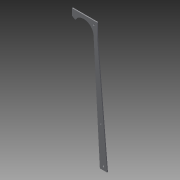
# Autodesk Inventor part: PassiveHooks2
Saved by Autodesk Inventor 2013 (Build 170138000, 138)
## iProperties
Created: 2013-02-07
Part Number: PassiveHooks2
Material: Generic
Document SubType Name: Sheet Metal
Designer: motoennies
Density: 1 g/cm^3
Sheet Metal Rule: Default
Author: motoennies
Autodesk Inventor part; units mm, degrees
ref_plane "YZ Plane" through (0, 0, 0) normal (1, 0, 0) x (0, 1, 0)
ref_plane "XZ Plane" through (0, 0, 0) normal (0, 1, 0) x (-1, 0, 0)
ref_plane "XY Plane" through (0, 0, 0) normal (0, 0, 1) x (1, 0, 0)
sketch "Sketch1" plane through (0, 0, 0) normal (0, 0, 1) x (1, 0, 0)
  arc A0 (34.8698, 1.9636) -> (-30.2459, 17.4625) centre (0, 0) ccw
  line L0 (-30.2459, 17.4625) -> (-41.2445, 23.8125)
  line L1 (0, 0) -> (-58.2409, 0) construction
  line L2 (47.853, -228.6) -> (34.8698, 1.9636)
  line L3 (82.55, -393.7) -> (47.4407, 4.1861)
  line L4 (57.15, -393.7) -> (82.55, -393.7)
  circle A1 centre (69.155, -381) radius 3.175
  line L5 (47.5493, 47.625) -> (47.5493, 2.9548)
  line L6 (-41.2445, 47.625) -> (-41.2445, 23.8125)
  line L7 (-41.2445, 47.625) -> (161.9555, 47.625) construction
  line L8 (-41.2445, 47.625) -> (161.9555, 47.625) construction
  line L9 (-41.2445, 47.625) -> (161.9555, 47.625) construction
  line L10 (-41.2445, 47.625) -> (161.9555, 47.625) construction
  line L11 (-41.2445, 47.625) -> (47.5493, 47.625)
  line L12 (47.853, -228.6) -> (57.15, -393.7)
  circle A2 centre (59.69, -255.905) radius 2.3813
  circle A3 centre (34.8493, 34.925) radius 3.175
  point P0 (47.5493, 25.2899)
  point P1 (51.4288, -292.1)
  dimension "d0" = 69.85
  dimension "d1" = 30
  dimension "d2" = 57.15
  dimension "d3" = 25.4
  dimension "d4" = 393.7
  dimension "d5" = 6.35
  dimension "d6" = 12.7
  dimension "d7" = 12.7
  dimension "d72" = 4.7625
  dimension "d73" = 2.54
  dimension "d74" = 137.795
  dimension "d76" = 6.35
  dimension "d77" = 12.7
  dimension "d78" = 12.7
  measures "d0" diameter of A0
  measures "d1" angle of L0 L1
  measures "d2" horizontal distance of L4.start point (0, 0)
  measures "d3" distance of L3.start L4.start
  measures "d4" distance from line of point (0, 0) L4
  measures "d5" diameter of A1
  measures "d6" distance from line of L4 A1.centre
  measures "d7" distance from line of L2 A1.centre
  measures "d72" diameter of A2
  measures "d73" horizontal distance of L4.start A2.centre
  measures "d74" distance from line of L4 A2.centre
  measures "d76" diameter of A3
  measures "d77" distance from line of L11 A3.centre
  measures "d78" horizontal distance of point (47.549, 25.29) A3.centre
extrude "Plate10" add sketch "Sketch1" along normal blind 3.175
equation "\"BendRadius\" = Thickness"
equation "\"BendReliefWidth\" = Thickness"
equation "\"BendReliefDepth\" = 0.5 * Thickness"
equation "\"CornerReliefSize\" = 4 * Thickness"
equation "\"MinimumRemnant\" = 2 * Thickness"
equation "\"TransitionRadius\" = BendRadius"
equation "\"JacobiRadiusSize\" = BendRadius"
equation "\"GapSize\" = Thickness"
equation "\"d10\" = BendRadius"
equation "\"d28\" = BendRadius"
equation "\"d71\" = BendRadius"
equation "\"d75\" = BendRadius"
equation "\"d79\" = BendRadius"
equation "\"Thickness\" = 3.175"
body "Solid5"
